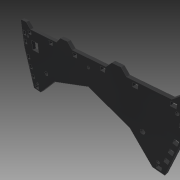
# Autodesk Inventor part: spool_stand_a
Saved by Autodesk Inventor 2014 (Build 180170000, 170)
## iProperties
Created: 2014-04-06
Part Number: spool_stand_a
Material: Plywood, Finish
Document SubType Name: Modeling
Designer: buben
Density: 0.552 g/cm^3
Appearance: Plywood - New
Author: buben
Autodesk Inventor part; units mm, degrees
ref_plane "YZ Plane" through (0, 0, 0) normal (1, 0, 0) x (0, 1, 0)
ref_plane "XZ Plane" through (0, 0, 0) normal (0, 1, 0) x (-1, 0, 0)
ref_plane "XY Plane" through (0, 0, 0) normal (0, 0, 1) x (1, 0, 0)
sketch "Sketch1" plane through (0, 0, 0) normal (0, 1, 0) x (-1, 0, 0)
  line L0 (-77.5, -76.6062) -> (-157.5, -47.4885)
  line L1 (-157.5, -47.4885) -> (-237.5, -76.6062)
  line L2 (-77.5, -76.6062) -> (-34.1062, -120)
  line L3 (-237.5, -76.6062) -> (-280.8938, -120)
  circle A0 centre (-157.5, -172.5) radius 132.5 construction
  line L4 (-280.8938, -120) -> (-300.8938, -120)
  line L5 (-34.1062, -120) -> (-14.1062, -120)
  circle A1 centre (-57.0709, -70) radius 11 construction
  circle A2 centre (-257.9291, -70) radius 11 construction
  line L6 (-14.1062, -120) -> (0, -40)
  line L7 (0, -40) -> (0, 0)
  line L8 (0, 0) -> (-315, 0)
  line L9 (-315, 0) -> (-315, -40)
  line L10 (-315, -40) -> (-300.8938, -120)
  circle A3 centre (-57.0709, -70) radius 4.1
  circle A4 centre (-257.9291, -70) radius 4.1
  dimension "d0" = 140
  dimension "d1" = 90
  dimension "d2" = 160
  dimension "d3" = 265
  dimension "d4" = 20
  dimension "d5" = 22
  dimension "d6" = 40
  dimension "d7" = 10
  dimension "d8" = 10
  dimension "d9" = 80
  dimension "d10" = 172.5
  dimension "d11" = 315
  dimension "d12" = 8.2
  dimension "d13" = 70
  constraints: 22 end point, 5 centre point, 4 horizontal alignment, 3 equal length, 3 perpendicular, 2 coincident, 2 equal radius, 2 tangent, 1 collinear, 1 horizontal, 1 vertical alignment
  measures "d0" angle of L1 L0
  measures "d1" angle of L3 L2
  measures "d2" distance of L1.end L0.start
  measures "d3" diameter of A0
  measures "d4" distance of L2.end L5.end
  measures "d5" diameter of A1
  measures "d6" distance of L6.end L7.end
  measures "d7" angle of L7 L6
  measures "d8" angle of L10 L9
  measures "d9" distance from line of L6.end L5
  measures "d10" distance from line of L8 A0.centre
  measures "d11" distance of L7.end L8.end
  measures "d12" diameter of A3
  measures "d13" distance from line of L8 A1.centre
extrude "Extrusion1" add sketch "Sketch1" along normal blind 6.5
sketch "Sketch4" plane through (0, 6.5, 0) normal (0, 1, 0) x (1, 0, 0)
  line L0 (0, 40) -> (0, 0) projected
  line L1 (0, 0) -> (315, 0) projected
  line L2 (315, 0) -> (315, 40) projected
  line L3 (34.1062, 120) -> (14.1062, 120) projected
  line L4 (14.1062, 120) -> (0, 40) projected
  line L5 (9.5, 9.5) -> (305.5, 9.5) construction
  line L6 (305.5, 9.5) -> (305.5, 3) construction
  line L7 (305.5, 3) -> (9.5, 3) construction
  line L8 (9.5, 3) -> (9.5, 9.5) construction
  line L9 (15.301, 117) -> (34.1062, 117) construction
  line L10 (34.1062, 117) -> (34.1062, 110.5) construction
  line L11 (34.1062, 110.5) -> (15.301, 110.5) construction
  line L12 (15.301, 110.5) -> (15.301, 117) construction
  line L13 (3, 40) -> (9.5, 40) construction
  line L14 (9.5, 40) -> (9.5, 0) construction
  line L15 (9.5, 0) -> (3, 0) construction
  line L16 (3, 0) -> (3, 40) construction
  line L17 (15.301, 109.5) -> (21.7023, 108.3713) construction
  line L18 (21.7023, 108.3713) -> (9.8229, 41) construction
  line L19 (9.8229, 41) -> (3.4216, 42.1287) construction
  line L20 (3.4216, 42.1287) -> (15.301, 109.5) construction
  line L21 (157.5, 47.4885) -> (157.5, 0) construction
  line L22 (17.5, 9.5) -> (25.5, 9.5)
  line L23 (25.5, 9.5) -> (25.5, 3)
  line L24 (25.5, 3) -> (17.5, 3)
  line L25 (17.5, 3) -> (17.5, 9.5)
  line L26 (71.9, 9.5) -> (79.9, 9.5)
  line L27 (79.9, 9.5) -> (79.9, 3)
  line L28 (79.9, 3) -> (71.9, 3)
  line L29 (71.9, 3) -> (71.9, 9.5)
  line L30 (126.3, 9.5) -> (134.3, 9.5)
  line L31 (134.3, 9.5) -> (134.3, 3)
  line L32 (134.3, 3) -> (126.3, 3)
  line L33 (126.3, 3) -> (126.3, 9.5)
  line L34 (3, 32) -> (9.5, 32)
  line L35 (9.5, 32) -> (9.5, 24)
  line L36 (9.5, 24) -> (3, 24)
  line L37 (3, 24) -> (3, 32)
  line L38 (3, 16) -> (9.5, 16)
  line L39 (9.5, 16) -> (9.5, 8)
  line L40 (9.5, 8) -> (3, 8)
  line L41 (3, 8) -> (3, 16)
  line L42 (20.7036, 117) -> (28.7036, 117)
  line L43 (28.7036, 117) -> (28.7036, 110.5)
  line L44 (28.7036, 110.5) -> (20.7036, 110.5)
  line L45 (20.7036, 110.5) -> (20.7036, 117)
  line L46 (13.3731, 98.566) -> (19.7743, 97.4373)
  line L47 (19.7743, 97.4373) -> (18.3851, 89.5588)
  line L48 (18.3851, 89.5588) -> (11.9839, 90.6876)
  line L49 (11.9839, 90.6876) -> (13.3731, 98.566)
  line L50 (10.0559, 79.7536) -> (16.4572, 78.6249)
  line L51 (16.4572, 78.6249) -> (15.068, 70.7464)
  line L52 (15.068, 70.7464) -> (8.6667, 71.8751)
  line L53 (8.6667, 71.8751) -> (10.0559, 79.7536)
  line L54 (6.7388, 60.9412) -> (13.14, 59.8124)
  line L55 (13.14, 59.8124) -> (11.7508, 51.934)
  line L56 (11.7508, 51.934) -> (5.3496, 53.0627)
  line L57 (5.3496, 53.0627) -> (6.7388, 60.9412)
  line L58 (9.9394, 60.3768) -> (11.8673, 71.3108) construction
  line L59 (8.5502, 52.4983) -> (6.6223, 41.5644) construction
  line L60 (13.2565, 79.1892) -> (15.1845, 90.1232) construction
  line L61 (16.5737, 98.0017) -> (18.5016, 108.9356) construction
  line L62 (6.25, 40) -> (6.25, 32) construction
  line L63 (6.25, 24) -> (6.25, 16) construction
  line L64 (6.25, 8) -> (6.25, 0) construction
  line L65 (25.5, 6.25) -> (71.9, 6.25) construction
  line L66 (79.9, 6.25) -> (126.3, 6.25) construction
  line L67 (134.3, 6.25) -> (180.7, 6.25) construction
  line L68 (297.5, 9.5) -> (289.5, 9.5)
  line L69 (289.5, 9.5) -> (289.5, 3)
  line L70 (289.5, 3) -> (297.5, 3)
  line L71 (297.5, 3) -> (297.5, 9.5)
  line L72 (243.1, 9.5) -> (235.1, 9.5)
  line L73 (235.1, 9.5) -> (235.1, 3)
  line L74 (235.1, 3) -> (243.1, 3)
  line L75 (243.1, 3) -> (243.1, 9.5)
  line L76 (188.7, 9.5) -> (180.7, 9.5)
  line L77 (180.7, 9.5) -> (180.7, 3)
  line L78 (180.7, 3) -> (188.7, 3)
  line L79 (188.7, 3) -> (188.7, 9.5)
  line L80 (312, 32) -> (305.5, 32)
  line L81 (305.5, 32) -> (305.5, 24)
  line L82 (305.5, 24) -> (312, 24)
  line L83 (312, 24) -> (312, 32)
  line L84 (312, 16) -> (305.5, 16)
  line L85 (305.5, 16) -> (305.5, 8)
  line L86 (305.5, 8) -> (312, 8)
  line L87 (312, 8) -> (312, 16)
  line L88 (294.2964, 117) -> (286.2964, 117)
  line L89 (286.2964, 117) -> (286.2964, 110.5)
  line L90 (286.2964, 110.5) -> (294.2964, 110.5)
  line L91 (294.2964, 110.5) -> (294.2964, 117)
  line L92 (301.6269, 98.566) -> (295.2257, 97.4373)
  line L93 (295.2257, 97.4373) -> (296.6149, 89.5588)
  line L94 (296.6149, 89.5588) -> (303.0161, 90.6876)
  line L95 (303.0161, 90.6876) -> (301.6269, 98.566)
  line L96 (304.9441, 79.7536) -> (298.5428, 78.6249)
  line L97 (298.5428, 78.6249) -> (299.932, 70.7464)
  line L98 (299.932, 70.7464) -> (306.3333, 71.8751)
  line L99 (306.3333, 71.8751) -> (304.9441, 79.7536)
  line L100 (308.2612, 60.9412) -> (301.86, 59.8124)
  line L101 (301.86, 59.8124) -> (303.2492, 51.934)
  line L102 (303.2492, 51.934) -> (309.6504, 53.0627)
  line L103 (309.6504, 53.0627) -> (308.2612, 60.9412)
  circle A0 centre (27.3023, 104.9) radius 2.6
  circle A1 centre (15.1, 15.1) radius 2.6
  circle A2 centre (157.5, 15.1) radius 2.6
  circle A3 centre (287.6977, 104.9) radius 2.6
  circle A4 centre (299.9, 15.1) radius 2.6
  point P0 (24.7036, 117)
  point P1 (24.7036, 117)
  point P2 (157.5, 6.25)
  point P3 (290.2964, 117)
  point P4 (290.2964, 117)
  point P5 (305.0606, 60.3768)
  point P6 (303.1327, 71.3108)
  point P7 (306.4498, 52.4983)
  point P8 (301.7435, 79.1892)
  point P9 (299.8155, 90.1232)
  point P10 (298.4263, 98.0017)
  point P11 (296.4984, 108.9356)
  point P12 (308.75, 32)
  point P13 (308.75, 24)
  point P14 (308.75, 16)
  point P15 (308.75, 8)
  point P16 (289.5, 6.25)
  point P17 (243.1, 6.25)
  point P18 (235.1, 6.25)
  point P19 (188.7, 6.25)
  dimension "d17" = 9.5
  dimension "d18" = 3
  dimension "d19" = 6.5
  dimension "d20" = 3
  dimension "d21" = 3
  dimension "d23" = 1
  dimension "d24" = 1
  dimension "d25" = 3
  dimension "d26" = 8
  dimension "d27" = 8
  dimension "d28" = 5.2
  dimension "d29" = 5.6
  dimension "d30" = 5.6
  dimension "d31" = 5.6
  dimension "d32" = 5.6
  constraints: 198 end point, 55 symmetric about line, 45 equal length, 23 midpoint, 20 collinear, 17 perpendicular, 9 horizontal, 5 centre point, 2 equal radius, 2 horizontal alignment, 2 point on line, 2 vertical alignment, 1 coincident, 2 other
  measures "d17" distance between parallel lines of L2 L6
  measures "d18" distance between parallel lines of L1 L7
  measures "d19" distance of L7.end L5.start
  measures "d20" distance between parallel lines of L3 L9
  measures "d21" distance between parallel lines of L4 L20
  measures "d23" distance from line of L13 L18.end
  measures "d24" distance from line of L11 L17.start
  measures "d25" distance between parallel lines of L0 L16
  measures "d26" distance of L22.start L22.end
  measures "d27" distance between parallel lines of L8 L25
  measures "d28" diameter of A2
  measures "d29" distance from line of L5 A2.centre
  measures "d30" distance from line of L14 A1.centre
  measures "d31" distance from line of L11 A0.centre
  measures "d32" horizontal distance of L17.end A0.centre
extrude "Extrusion2" cut sketch "Sketch4" against normal through all
sketch "Sketch5" plane through (0, 6.5, 0) normal (0, 1, 0) x (1, 0, 0)
  line L0 (0, 0) -> (315, 0) projected
  line L1 (34.1062, 120) -> (14.1062, 120) projected
  line L2 (0, 0) -> (0, -10)
  line L3 (0, -10) -> (15, -10)
  line L4 (15, -10) -> (25, 0)
  line L5 (25, 0) -> (0, 0)
  line L6 (90, 0) -> (100, -10)
  line L7 (100, -10) -> (115, -10)
  line L8 (115, -10) -> (125, 0)
  line L9 (125, 0) -> (90, 0)
  line L10 (190, 0) -> (200, -10)
  line L11 (200, -10) -> (215, -10)
  line L12 (215, -10) -> (225, 0)
  line L13 (315, 0) -> (315, -10)
  line L14 (315, -10) -> (300, -10)
  line L15 (300, -10) -> (290, 0)
  line L16 (20, -5) -> (95, -5) construction
  line L17 (120, -5) -> (195, -5) construction
  line L18 (220, -5) -> (295, -5) construction
  dimension "d35" = 10
  dimension "d36" = 45
  dimension "d37" = 15
  dimension "d38" = 15
  dimension "d39" = 15
  dimension "d40" = 15
  constraints: 34 end point, 9 perpendicular, 7 collinear, 6 midpoint, 6 point on line, 2 parallel
  measures "d35" distance of L0.start L2.end
  measures "d36" angle of L5 L4
  measures "d37" distance of L2.end L3.end
  measures "d38" distance of L6.end L7.end
  measures "d39" distance of L10.end L11.end
  measures "d40" distance of L13.end L14.end
extrude "Extrusion3" add sketch "Sketch5" against normal blind 6.5
chamfer "Chamfer1" distance 2 angle 45 2 edges at (0, 3.25, 10) (315, 3.25, 10)
sketch "Sketch6" plane through (0, 6.5, 0) normal (0, 1, 0) x (1, 0, 0)
  line L0 (71.9, 9.5) -> (79.9, 9.5) projected
  line L1 (9.5, 32) -> (9.5, 24) projected
  line L2 (24.5, 37) -> (41, 37)
  line L3 (41, 37) -> (41, 19.5)
  line L4 (41, 19.5) -> (24.5, 19.5)
  line L5 (24.5, 19.5) -> (24.5, 37)
  point P0 (0, 0)
  dimension "d46" = 17.5
  dimension "d47" = 16.5
  dimension "d48" = 10
  dimension "d49" = 15
  constraints: 8 end point, 2 parallel, 1 horizontal, 1 perpendicular
  measures "d46" distance of L4.end L2.start
  measures "d47" distance of L3.end L4.end
  measures "d48" distance between parallel lines of L0 L4
  measures "d49" distance between parallel lines of L1 L5
extrude "Extrusion4" cut sketch "Sketch6" against normal through all
equation "\"d8\" = d7"
equation "\"d17\" = d16 + d19"
equation "\"d18\" = d16"
equation "\"d31\" = d30"
equation "\"d32\" = d31"
equation "\"d38\" = d37"
equation "\"d39\" = d38"
equation "\"d40\" = d39"
equation "\"d16\" = 3"
body "Solid1"
